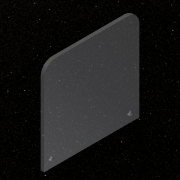
# Autodesk Inventor part: Divider
Saved by Autodesk Inventor 2012 (Build 160160000, 160)
## iProperties
Created: 2012-11-14
Part Number: Divider
Material: Default
Document SubType Name: Modeling
Designer: SONY
Density: 1 g/cm^3
Author: SONY
Autodesk Inventor part; units mm, degrees
ref_plane "YZ Plane" through (0, 0, 0) normal (1, 0, 0) x (0, 1, 0)
sketch "Sketch1" plane through (0, 0, 0) normal (0, 0, 1) x (1, 0, 0)
  line L0 (104.68, -86.36) -> (104.68, -10.7) projected
  line L1 (101.505, -86.36) -> (104.68, -86.36) projected
  line L2 (148.8666, 2) -> (0, 2) projected
  line L3 (0, 0) -> (171.285, 0) projected
  line L4 (104.68, -86.36) -> (101.505, -86.36)
  line L5 (101.505, -86.36) -> (101.505, 16.1032)
  line L6 (101.505, 16.1032) -> (104.68, 16.1032)
  line L7 (104.68, 16.1032) -> (104.68, -86.36)
  dimension "d0" = 3.175
  constraints: 8 end point, 2 parallel, 1 horizontal, 1 perpendicular
  measures "d0" distance between parallel lines of L7 L5
ref_plane "Work Plane1" through (98.965, -88.9, 88.0899) normal (0, 0, -1) x (0, 1, 0)
extrude "Extrusion1" add sketch "Sketch1" along normal up to surface (88.0899 mm away)
ref_plane "Work Plane2" through (0, 0, 90.0899) normal (-1, 0, 0) x (0, 0, 1)
sketch "Sketch2" plane through (0, 0, 90.0899) normal (-1, 0, 0) x (0, 0, 1)
  arc A0 (-79.3899, 2) -> (-92.0899, -10.7) centre (-79.3899, -10.7) ccw
  line L0 (-79.3899, 2) -> (-12.7, 2)
  arc A1 (0, -10.7) -> (-12.7, 2) centre (-12.7, -10.7) ccw
  line L1 (0, -10.7) -> (0, -82.9)
  arc A2 (0, -82.9) -> (2, -84.9) centre (2, -82.9) ccw
  line L2 (2, -84.9) -> (6.985, -84.9)
  line L3 (6.985, -84.9) -> (6.985, -88.9)
  line L4 (6.985, -88.9) -> (3.5017, -88.9)
  arc A3 (2.4019, -88.265) -> (3.5017, -88.9) centre (3.5017, -87.63) ccw
  arc A4 (2.4019, -88.265) -> (0.2021, -88.265) centre (1.302, -88.9) ccw
  arc A5 (-0.8977, -88.9) -> (0.2021, -88.265) centre (-0.8977, -87.63) ccw
  line L5 (-0.8977, -88.9) -> (-2, -88.9)
  line L6 (-2, -88.9) -> (-2, -10.7)
  arc A6 (-2, -10.7) -> (-12.7, 0) centre (-12.7, -10.7) ccw
  line L7 (-12.7, 0) -> (-79.3899, 0)
  arc A7 (-79.3899, 0) -> (-90.0899, -10.7) centre (-79.3899, -10.7) ccw
  line L8 (-90.0899, -10.7) -> (-90.0899, -88.9)
  line L9 (-90.0899, -88.9) -> (-91.1922, -88.9)
  arc A8 (-92.2921, -88.265) -> (-91.1922, -88.9) centre (-91.1922, -87.63) ccw
  arc A9 (-92.2921, -88.265) -> (-94.4918, -88.265) centre (-93.3919, -88.9) ccw
  arc A10 (-95.5916, -88.9) -> (-94.4918, -88.265) centre (-95.5916, -87.63) ccw
  line L10 (-95.5916, -88.9) -> (-99.0749, -88.9)
  line L11 (-99.0749, -88.9) -> (-99.0749, -84.9)
  line L12 (-99.0749, -84.9) -> (-94.0899, -84.9)
  arc A11 (-94.0899, -84.9) -> (-92.0899, -82.9) centre (-94.0899, -82.9) ccw
  line L13 (-92.0899, -82.9) -> (-92.0899, -10.7)
  line L14 (-2, -88.9) -> (-90.0899, -88.9)
  point P0 (-90.0899, 0)
  constraints: 30 end point, 24 point on circle, 12 centre point, 8 horizontal, 6 vertical, 1 perpendicular, 50 other
extrude "Extrusion2" cut sketch "Sketch2" against normal through all contours L8 A7 L7 A6 L6 L14 keep common part
sketch "Sketch3" plane through (101.505, -86.36, 0) normal (-1, 0, 0) x (0, 0, 1)
  line L0 (0, 0) -> (0, 75.66) projected
  line L1 (0, 0) -> (88.0899, 0) projected
  line L2 (88.0899, 75.66) -> (88.0899, 0) projected
  circle A0 centre (7.62, 6.35) radius 1.5875
  circle A1 centre (80.4699, 6.35) radius 1.5875
  line L3 (7.62, 6.35) -> (67.6256, 6.35) construction
  point P0 (0, 86.36)
  dimension "d5" = 3.175
  dimension "d6" = 3.175
  dimension "d7" = 6.35
  dimension "d9" = 7.62
  dimension "d10" = 7.62
  constraints: 2 centre point, 2 end point, 1 perpendicular, 1 point on line
  measures "d5" diameter of A0
  measures "d6" diameter of A1
  measures "d7" distance between parallel lines of L1 L3
  measures "d9" distance from line of L2 A1.centre
  measures "d10" distance from line of L0 L3.start
extrude "Extrusion3" cut sketch "Sketch3" against normal through all
equation "\"d10\" = d9"
body "Solid1"
